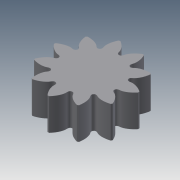
# Autodesk Inventor part: tilt-gear_A_test
Saved by Autodesk Inventor 2018 (Build 220112000, 112)
## iProperties
Created: 2019-02-28
Part Number: tilt-gear_A_test
Material: Generic
Document SubType Name: Modeling
Designer: Tsche
Density: 1 g/cm^3
Appearance: Default
Author: Tsche
Autodesk Inventor part; units mm, degrees
ref_plane "YZ Plane" through (0, 0, 0) normal (1, 0, 0) x (0, 1, 0)
ref_plane "XZ Plane" through (0, 0, 0) normal (0, 1, 0) x (-1, 0, 0)
ref_plane "XY Plane" through (0, 0, 0) normal (0, 0, 1) x (1, 0, 0)
sketch "Sketch2" plane through (0, 0, 0) normal (0, 0, 1) x (1, 0, 0)
  spline S0 degree 3 poles (-1.7687, 6.4561) (-1.7194, 6.4252) (-1.6209, 6.3634) (-1.4781, 6.263) (-1.3393, 6.1572) (-1.2053, 6.0454) (-1.0766, 5.9274) (-0.954, 5.8033) (-0.8381, 5.6727) (-0.73, 5.5357) (-0.6309, 5.3919) (-0.5574, 5.2664) (-0.5053, 5.1623) (-0.4702, 5.0824) (-0.4398, 5.0006) (-0.4158, 4.9166) (-0.4009, 4.8306) (-0.3753, 4.747) (-0.3419, 4.6663) (-0.3052, 4.6032) (-0.2699, 4.5569) (-0.24, 4.525) (-0.2067, 4.4967) (-0.1699, 4.473) (-0.1299, 4.4553) (-0.073, 4.4411) (0, 4.446) (0.073, 4.4411) (0.1299, 4.4553) (0.1699, 4.473) (0.2067, 4.4967) (0.24, 4.525) (0.2699, 4.5569) (0.3052, 4.6032) (0.3419, 4.6663) (0.3753, 4.747) (0.4009, 4.8306) (0.4158, 4.9166) (0.4398, 5.0006) (0.4702, 5.0824) (0.5053, 5.1623) (0.5574, 5.2664) (0.6309, 5.3919) (0.73, 5.5357) (0.8381, 5.6727) (0.954, 5.8033) (1.0766, 5.9274) (1.2053, 6.0454) (1.3393, 6.1572) (1.4781, 6.263) (1.6209, 6.3634) (1.7194, 6.4252) (1.7687, 6.4561) knots 0 0 0 0 0.017447 0.034893 0.05234 0.069787 0.087233 0.104679 0.122125 0.13957 0.157015 0.174458 0.183181 0.191904 0.200626 0.209347 0.21807 0.226792 0.235512 0.24423 0.248591 0.252953 0.257314 0.261674 0.266033 0.270392 0.279108 0.287825 0.292183 0.296543 0.300903 0.305264 0.309625 0.313987 0.322705 0.331425 0.340146 0.34887 0.35759 0.366313 0.375036 0.383759 0.401202 0.418647 0.436092 0.453538 0.470984 0.48843 0.505877 0.523323 0.54077 0.558217 0.558217 0.558217 0.558217
  circle A0 centre (0, 0) radius 4.444 construction
  circle A1 centre (0, 0) radius 4.8875 construction
  circle A2 centre (0, 0) radius 5.694 construction
  circle A3 centre (0, 0) radius 6.694
  point P0 (-1.6217, 6.3621)
  point P1 (-1.4787, 6.2621)
  point P2 (-1.3401, 6.1562)
  point P3 (-1.2062, 6.0444)
  point P4 (-1.0776, 5.9264)
  point P5 (-0.9551, 5.8022)
  point P6 (-0.8394, 5.6717)
  point P7 (-0.7315, 5.5346)
  point P8 (-0.6327, 5.3908)
  point P9 (-0.5449, 5.2401)
  point P10 (-0.506, 5.162)
  point P11 (-0.471, 5.0821)
  point P12 (-0.4409, 5.0002)
  point P13 (-0.4173, 4.9163)
  point P14 (-0.3991, 4.831)
  point P15 (-0.374, 4.7474)
  point P16 (-0.3401, 4.6671)
  point P17 (-0.2959, 4.592)
  point P18 (-0.2693, 4.5574)
  point P19 (-0.2395, 4.5256)
  point P20 (-0.2062, 4.4974)
  point P21 (-0.1694, 4.474)
  point P22 (-0.1295, 4.4565)
  point P23 (-0.0871, 4.4462)
  point P24 (0, 4.444)
  point P25 (0.0871, 4.4462)
  point P26 (0.1295, 4.4565)
  point P27 (0.1694, 4.474)
  point P28 (0.2062, 4.4974)
  point P29 (0.2395, 4.5256)
  point P30 (0.2693, 4.5574)
  point P31 (0.2959, 4.592)
  point P32 (0.3401, 4.6671)
  point P33 (0.374, 4.7474)
  point P34 (0.3991, 4.831)
  point P35 (0.4173, 4.9163)
  point P36 (0.4409, 5.0002)
  point P37 (0.471, 5.0821)
  point P38 (0.506, 5.162)
  point P39 (0.5449, 5.2401)
  point P40 (0.6327, 5.3908)
  point P41 (0.7315, 5.5346)
  point P42 (0.8394, 5.6717)
  point P43 (0.9551, 5.8022)
  point P44 (1.0776, 5.9264)
  point P45 (1.2062, 6.0444)
  point P46 (1.3401, 6.1562)
  point P47 (1.4787, 6.2621)
  point P48 (1.6217, 6.3621)
  constraints: 4 centre point, 2 point on circle, 107 other
extrude "Extrusion3" add sketch "Sketch2" along normal blind 5
extrude "Extrusion4" cut sketch "Sketch2" along normal blind 5 contours A3 S0 picked at (-0.1908, 5.807)
pattern_circular "Circular Pattern2" count 11 over 360 about axis through (0, 0, -10) along (0, 0, 1) of "Extrusion4"
body "Solid2"
